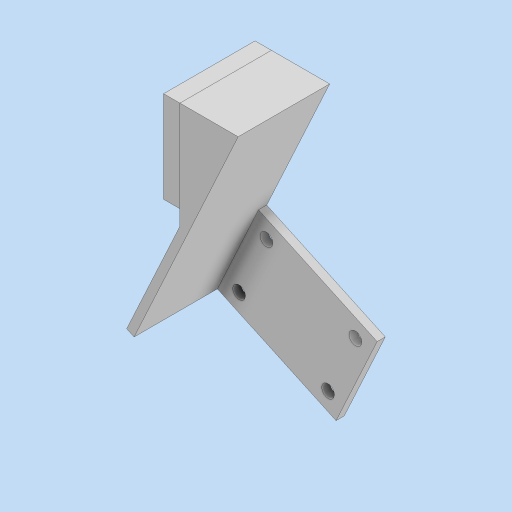
# Autodesk Inventor part: back mount
Saved by Autodesk Inventor 2024 (Build 280153000, 153)
## iProperties
Created: 2024-02-17
Part Number: back mount
Material: Generic
Document SubType Name: Modeling
Designer: mones
Density: 1 g/cm^3
Appearance: Default
Author: mones
Autodesk Inventor part; units mm, degrees
ref_plane "YZ Plane" through (0, 0, 0) normal (1, 0, 0) x (0, 1, 0)
ref_plane "XZ Plane" through (0, 0, 0) normal (0, 1, 0) x (-1, 0, 0)
ref_plane "XY Plane" through (0, 0, 0) normal (0, 0, 1) x (1, 0, 0)
sketch "Sketch1" plane through (0, 0, 0) normal (1, 0, 0) x (0, 1, 0)
  line L0 (-12.2044, 14.0187) -> (-12.2044, -21.5388)
  line L1 (-12.2044, -21.5388) -> (-21.2212, -21.5388)
  line L2 (-21.2212, -16.1112) -> (-21.2212, 10.4119)
  line L3 (-21.2212, 14.0187) -> (-12.2044, 14.0187)
  line L4 (-47.769, -16.1112) -> (-47.769, -21.5388)
  line L5 (-47.769, -21.5388) -> (-44.4011, -21.5388)
  line L6 (-47.769, -16.1112) -> (-47.769, 14.0187)
  line L7 (-47.769, 14.0187) -> (-44.4011, 14.0187)
  line L8 (-44.4011, 10.4119) -> (-44.4011, -16.1112)
  line L9 (-21.2212, -16.1112) -> (-21.2212, -21.5388)
  line L10 (-44.4011, -16.1112) -> (-44.4011, -21.5388)
  line L11 (-21.2212, 10.4119) -> (-44.4011, 10.4119)
  line L12 (-44.4011, 14.0187) -> (-21.2212, 14.0187)
  constraints: 26 end point, 4 parallel, 4 perpendicular, 1 point on line, 1 vertical
extrude "Extrusion1" add sketch "Sketch1" along normal blind 6.35
sketch "Sketch3" plane through (0, -21.2212, -21.5388) normal (0, 0, -1) x (-1, 0, 0)
  line L0 (-6.3501, 9.0172) -> (-6.3501, -26.5428)
  line L1 (-6.3501, -26.5428) -> (-6.3501, -32.4404)
  line L2 (-6.3501, -32.4404) -> (14.3519, -77.2848)
  line L3 (-6.3501, -32.4404) -> (43.0421, -32.4404) construction
  line L4 (-6.3501, 9.0172) -> (-28.9857, 9.0172)
  line L5 (14.3519, -77.2848) -> (11.4692, -78.6156)
  line L6 (11.4692, -78.6156) -> (-28.9857, 9.0172)
  dimension "d29" = 96.52
  dimension "d30" = 22.6355
  dimension "d31" = 35.56
  constraints: 14 end point, 2 horizontal, 2 vertical, 1 equal length, 1 perpendicular
  measures "d29" distance of L5.end L4.end
  measures "d30" distance of L0.start L4.end
  measures "d31" distance of L0.start L0.end
extrude "Extrusion2" add sketch "Sketch3" against normal blind 35.56
sketch "Sketch4" plane through (0, -21.2212, -21.5388) normal (0, 0, -1) x (-1, 0, 0)
  line L0 (11.4705, -78.6183) -> (-34.652, -99.9104)
  line L1 (11.4705, -78.6183) -> (62.2705, -78.6183) construction
  line L2 (-34.652, -99.9104) -> (-50.6211, -65.3185)
  line L3 (-50.6211, -65.3185) -> (-4.4986, -44.0264)
  line L4 (-4.4986, -44.0264) -> (11.4705, -78.6183)
  line L5 (-50.6211, -65.3185) -> (-47.3708, -72.3592)
  circle A0 centre (-42.1943, -68.4223) radius 2.4892
  circle A1 centre (-7.6024, -52.4532) radius 2.4892
  circle A2 centre (3.0437, -75.5145) radius 2.4892
  circle A3 centre (-31.5482, -91.4835) radius 2.4892
  dimension "d15" = 50.8
  dimension "d16" = 155.22
  dimension "d17" = 38.1
  dimension "d25" = 4.9784
  dimension "d26" = 4.9784
  dimension "d27" = 4.9784
  dimension "d28" = 4.9784
  dimension "d32" = 6.35
  dimension "d34" = 6.35
  dimension "d35" = 6.35
  dimension "d37" = 6.35
  dimension "d38" = 6.35
  dimension "d40" = 6.35
  dimension "d42" = 6.35
  dimension "d44" = 6.35
  constraints: 12 end point, 4 centre point, 3 perpendicular, 1 equal length, 1 horizontal, 1 point on line
  measures "d15" distance of L0.start L0.end
  measures "d16" angle of L0 L1
  measures "d17" distance of L0.end L2.end
  measures "d25" diameter of A0
  measures "d26" diameter of A1
  measures "d27" diameter of A2
  measures "d28" diameter of A3
  measures "d32" distance from line of A1.centre L3
  measures "d34" distance from line of A1.centre L4
  measures "d35" distance from line of A2.centre L4
  measures "d37" distance from line of A2.centre L0
  measures "d38" distance from line of A3.centre L0
  measures "d40" distance from line of A3.centre L2
  measures "d42" distance from line of A0.centre L3
  measures "d44" distance from line of L2 A0.centre
extrude "Extrusion3" add sketch "Sketch4" against normal blind 3.175
body "Solid1"
